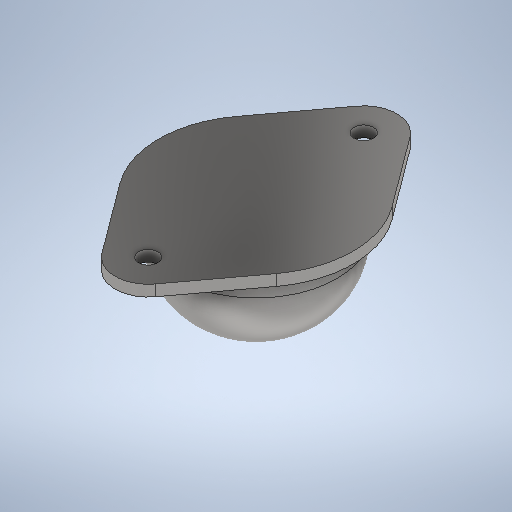
# Autodesk Inventor part: roulette
Saved by Autodesk Inventor 2025 (Build 290162000, 162)
## iProperties
Created: 2024-09-13
Part Number: roulette
Material: Générique
Document SubType Name: Modeling
Designer: chass
Density: 1 g/cm^3
Appearance: Par défaut
Author: chass
Autodesk Inventor part; units mm, degrees
ref_plane "YZ Plane" through (0, 0, 0) normal (1, 0, 0) x (0, 1, 0)
ref_plane "XZ Plane" through (0, 0, 0) normal (0, 1, 0) x (-1, 0, 0)
ref_plane "XY Plane" through (0, 0, 0) normal (0, 0, 1) x (1, 0, 0)
sketch "Esquisse1" plane through (0, 0, 0) normal (0, 1, 0) x (-1, 0, 0)
  circle A0 centre (0, 0) radius 17.5
  circle A1 centre (0, 19.4) radius 1.75
  line L0 (13, 0) -> (-12, 0)
  circle A2 centre (0, -19.4) radius 1.75
  circle A3 centre (0, 19.4) radius 5.9464
  line L1 (4.7769, 22.9414) -> (14.0581, 10.422)
  line L2 (0, 31) -> (0, -30)
  line L3 (-4.7769, 22.9414) -> (-14.0581, 10.422)
  circle A4 centre (0, -19.4) radius 5.9464
  line L4 (4.7769, -22.9414) -> (14.0581, -10.422)
  line L5 (-4.7769, -22.9414) -> (-14.0581, -10.422)
  dimension "d1" = 35
  dimension "d3" = 11.8928
  dimension "d0" = 3.5
  dimension "d2" = 19.4
  constraints: 12 end point, 8 symmetric about line, 3 point on line, 2 centre point, 2 coincident, 2 horizontal, 1 vertical, 12 other
  measures "d0" diameter of A1
  measures "d2" distance from line of L0 A1.centre
extrude "Extrusion1" add sketch "Esquisse1" along normal blind 2 contours A0 A4 L2 A3 | A0 A3 L1 | L4 A4 A0 | A3 L2 A0 | A0 L2 A1 A3 | A4 L2 A2 A0 | A0 L2 A4 | L2 A3 A0 | A0 A3 L2 A1 | L2 A4 A0 A3 | L2 A2 A4 A0 | A0 A4 L2 | A0 L3 A3 | A4 L5 A0
sketch "Esquisse2" plane through (0, 0, 0) normal (0, -1, 0) x (1, 0, 0)
  circle A0 centre (0, 0) radius 14.5602
  constraints: 1 centre point, 1 coincident
extrude "Extrusion2" add sketch "Esquisse2" along normal blind 17
fillet "Congé1" radius 13.25 1 edges at (-14.5602, -17, 0)
